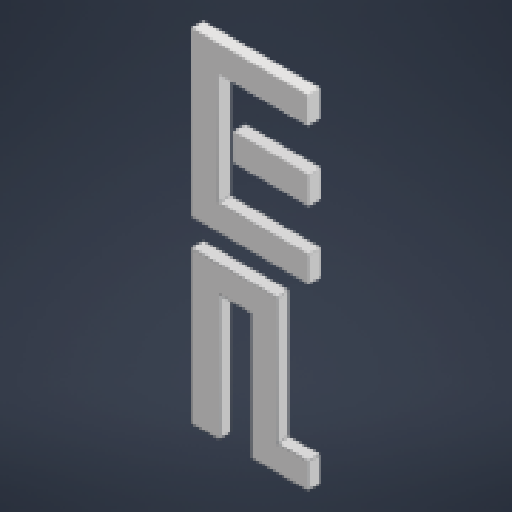
# Autodesk Inventor part: ROBOILO LOGO
Saved by Autodesk Inventor 2024 (Build 280153000, 153)
## iProperties
Created: 2024-06-09
Part Number: ROBOILO LOGO
Material: Generic
Document SubType Name: Modeling
Designer: mateu
Density: 1 g/cm^3
Appearance: Default
Author: mateu
Autodesk Inventor part; units mm, degrees
ref_plane "YZ Plane" through (0, 0, 0) normal (1, 0, 0) x (0, 1, 0)
ref_plane "XZ Plane" through (0, 0, 0) normal (0, 1, 0) x (-1, 0, 0)
ref_plane "XY Plane" through (0, 0, 0) normal (0, 0, 1) x (1, 0, 0)
sketch "Sketch1" plane through (0, 0, 0) normal (0, 0, 1) x (1, 0, 0)
  line L0 (-26.5523, -13.8097) -> (-23.4761, -13.8097) projected
  line L1 (-26.5523, -1.2089) -> (-26.5523, -13.8097) projected
  line L2 (-35.1023, -1.2089) -> (-26.5523, -1.2089) projected
  line L3 (-35.1023, -16.3589) -> (-35.1023, -1.2089) projected
  line L4 (-32.3273, -16.3589) -> (-35.1023, -16.3589) projected
  line L5 (-32.3273, -3.8452) -> (-32.3273, -16.3589) projected
  line L6 (-29.0999, -3.8452) -> (-32.3273, -3.8452) projected
  line L7 (-29.0999, -16.3589) -> (-29.0999, -3.8452) projected
  line L8 (-23.4761, -16.3589) -> (-29.0999, -16.3589) projected
  line L9 (-23.4761, -13.8097) -> (-23.4761, -16.3589) projected
  line L10 (-32.4023, 4.0411) -> (-23.4023, 4.0411) projected
  line L11 (-32.4023, 15.1366) -> (-32.4023, 4.0411) projected
  line L12 (-23.4769, 15.1366) -> (-32.4023, 15.1366) projected
  line L13 (-23.4769, 17.7661) -> (-23.4769, 15.1366) projected
  line L14 (-35.1023, 17.7661) -> (-23.4769, 17.7661) projected
  line L15 (-35.1023, 1.4911) -> (-35.1023, 17.7661) projected
  line L16 (-23.4023, 1.4911) -> (-35.1023, 1.4911) projected
  line L17 (-23.4023, 4.0411) -> (-23.4023, 1.4911) projected
  line L18 (-30.9023, 8.2411) -> (-30.9023, 10.9411) projected
  line L19 (-23.4023, 8.2411) -> (-30.9023, 8.2411) projected
  line L20 (-23.4023, 10.9411) -> (-23.4023, 8.2411) projected
  line L21 (-30.9023, 10.9411) -> (-23.4023, 10.9411) projected
  point P0 (0, 0)
extrude "Extrusion1" add sketch "Sketch1" along normal blind 1.2
body "Solid1"
